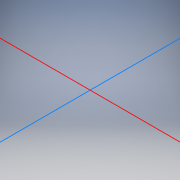
# Autodesk Inventor part: encoder
Saved by Autodesk Inventor 2022 (Build 260153000, 153)
## iProperties
Created: 2022-11-07
Part Number: encoder
Material: Типовые
Document SubType Name: Modeling
Designer: Petrov Ivan
Density: 1 g/cm^3
Appearance: По умолчанию
Author: Petrov Ivan
Autodesk Inventor part; units mm, degrees
ref_plane "YZ Plane" through (0, 0, 0) normal (1, 0, 0) x (0, 1, 0)
ref_plane "XZ Plane" through (0, 0, 0) normal (0, 1, 0) x (-1, 0, 0)
ref_plane "XY Plane" through (0, 0, 0) normal (0, 0, 1) x (1, 0, 0)
sketch "Эскиз1" plane through (0, 0, 0) normal (0, 1, 0) x (-1, 0, 0)
  circle A0 centre (0, 0) radius 16
  line L0 (15.5, 3.9686) -> (15.5, -3.9686)
  line L1 (-15.5, 3.9686) -> (-15.5, -3.9686)
  dimension "d0" = 32
  dimension "d1" = 15.5
  dimension "d2" = 15.5
  constraints: 4 end point, 4 point on circle, 1 centre point, 1 coincident, 1 parallel, 1 vertical
  measures "d0" diameter of A0
  measures "d1" distance from line of point (0, 0) L0
  measures "d2" distance from line of L1 point (0, 0)
extrude "Выдавливание1" add sketch "Эскиз1" along normal blind 2 contours L0 A0 L1
sketch "Эскиз2" plane through (0, 2, 0) normal (0, 1, 0) x (1, 0, 0)
  circle A0 centre (0, 0) radius 1
  dimension "d5" = 2
  constraints: 1 centre point, 1 coincident
  measures "d5" diameter of A0
extrude "Выдавливание2" add sketch "Эскиз2" along normal blind 7
ref_plane "РабПлоскость1" through (0, 8.4, 0) normal (0, 1, 0) x (1, 0, 0)
sketch "Эскиз3" plane through (0, 8.4, 0) normal (0, 1, 0) x (1, 0, 0)
  circle A0 centre (0, 0) radius 1 projected
  circle A1 centre (0, 0) radius 6.5
  dimension "d9" = 13
  constraints: 1 centre point, 1 coincident
  measures "d9" diameter of A1
extrude "Выдавливание3" add sketch "Эскиз3" against normal blind 5
fillet "Сопряжение1" radius 0.3 2 edges at (-6.5, 8.4, 0) (-6.5, 3.4, 0)
equation "\"d2\" = d1"
